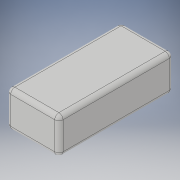
# Autodesk Inventor part: battery
Saved by Autodesk Inventor 2018 (Build 220112000, 112)
## iProperties
Created: 2018-05-07
Part Number: battery
Material: Generic
Document SubType Name: Modeling
Designer: mmarkle
Density: 1 g/cm^3
Appearance: Default
Author: mmarkle
Autodesk Inventor part; units mm, degrees
ref_plane "YZ Plane" through (0, 0, 0) normal (1, 0, 0) x (0, 1, 0)
ref_plane "XZ Plane" through (0, 0, 0) normal (0, 1, 0) x (-1, 0, 0)
ref_plane "XY Plane" through (0, 0, 0) normal (0, 0, 1) x (1, 0, 0)
sketch "Sketch1" plane through (0, 0, 0) normal (0, 1, 0) x (-1, 0, 0)
  line L0 (-16, 35) -> (16, 35)
  line L1 (16, 35) -> (16, -35)
  line L2 (16, -35) -> (-16, -35)
  line L3 (-16, -35) -> (-16, 35)
  line L4 (-16, 35) -> (16, -35) construction
  line L5 (16, 35) -> (-16, -35) construction
  point P0 (0, 0)
  dimension "d0" = 32
  dimension "d1" = 70
  constraints: 12 end point, 2 midpoint, 2 parallel, 1 horizontal, 1 perpendicular
  measures "d0" distance of L1.end L2.end
  measures "d1" distance of L0.end L1.end
extrude "Extrusion1" add sketch "Sketch1" along normal blind 22
fillet "Fillet1" radius 2.54 12 edges at (-16, 0, 0) (-16, 11, 35) (-16, 22, 0) (-16, 11, -35) (0, 0, -35) (0, 22, -35) (16, 11, -35) (16, 0, 0) (16, 22, 0) (16, 11, 35) (0, 0, 35) (0, 22, 35)
body "Solid1"
